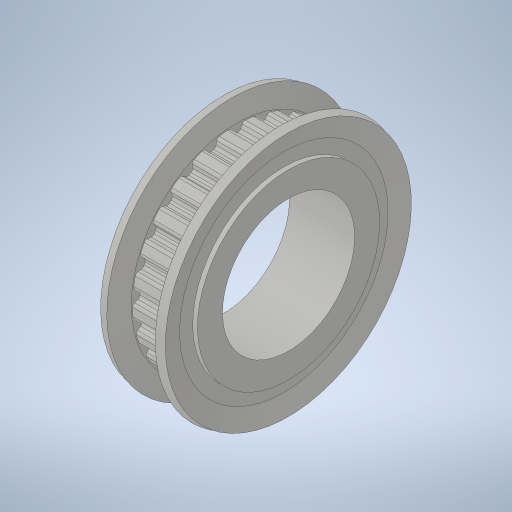
# Autodesk Inventor part: ATP25XL025-A-HUK_a
Saved by Autodesk Inventor 2023.1 (Build 271208000, 208)
## iProperties
Created: 2022-11-04
Part Number: ATP25XL025-A-HUK_a
Material: Generic
Catalog Web Link: www.cadenas.de
Description: ATP_ _XL025, ATP_ _XL031, ATP_ _ XL037, ATP_ _XL050, BTP_ _XL025, BTP_ _XL031, BTP_ _XL037, BTP_ _XL050, KTP_ _XL025, KTP_ _XL031, KTP_ _ XL037, KTP_ _XL050, NTP_ _XL025, NTP_ _XL031, NTP_ _ XL037, NTP_ _XL050, MTP_ _XL025, MTP_ _ XL037, MTP_ _XL050, MTPB_ _XL025, MTPB_ _ XL037, MTPB_ _XL050, MTPP_ _XL025, MTPP_ _ XL037, MTPP_ _XL050, STP_ _XL025, STP_ _ XL037, STP_ _XL050_aI-Timing Pulleys XL Type
Vendor: MISUMI
Document SubType Name: Modeling
Designer: psAdmin
Manufacturer: MISUMI
Mass: 10.0288 g
Surface Area: 66.7014 cm^2
Volume: 10.0288 cm^3
Density: 1 g/cm^3
Appearance: PSOLRGB-175-175-175
Category: PARTsolutions
Company: MISUMI
PSOL_IDENT_0: {$CADENAS_DATA/23d-libs/misumi/metric/51_timing_pulleys/timing_pulleys_inch/atp_xl_inch.prj},697 {VT
PSOL_IDENT_1: YP=3D},{NB=ATP25XL025-A-HUK_a},{LINA=ATP25XL025-A-HUK},{NN=ATP_ _XL025, ATP_ _XL031, ATP_ _ XL037, A
PSOL_IDENT_2: TP_ _XL050, BTP_ _XL025, BTP_ _XL031, BTP_ _XL037, BTP_ _XL050, KTP_ _XL025, KTP_ _XL031, KTP_ _ XL0
PSOL_IDENT_3: 37, KTP_ _XL050, NTP_ _XL025, NTP_ _XL031, NTP_ _ XL037, NTP_ _XL050, MTP_ _XL025, MTP_ _ XL037, MTP
PSOL_IDENT_4: _ _XL050, MTPB_ _XL025, MTPB_ _ XL037, MTPB_ _XL050, MTPP_ _XL025, MTPP_ _ XL037, MTPP_ _XL050, STP_
PSOL_IDENT_5: _XL025, STP_ _ XL037, STP_ _XL050_aI},{DATE=08.06.2021 06:34:01},{GEOMDATE=19.11.2018 09:46:42},{VE
PSOL_IDENT_6: RSION=},{LINEID=120},{WBVAR=MATP,ST,TNW,PS,SHS,DD,ALT2,M,QSC,QFC,QTC,ALT7,K,KSC,KFC,KTC,ALT1,ALT3,AL
PSOL_IDENT_7: T4,ALT5,FC,ALT6,TPC,ALT8,BC,ALT9,SLH},{WBNUMERIC=DD,QSC,QFC,QTC,K,KSC,KFC,KTC,FC,TPC,BC,SLH}  {NB=AT
PSOL_IDENT_8: P25XL025-A-HUK_a},{LINA=ATP25XL025-A-HUK},{KT=DUMMY},{PN=ATP25XL025-A-HUK},{TYPE=ATP},{MATP=ATP},{MA
PSOL_IDENT_9: TPA='ATP','2017 Aluminum Alloy (Duralumin)','MTP','1045 Carbon Steel','STP','304 Stainless Steel'},{
PSOL_IDENT_10: MATF=5052 Aluminum Alloy},{ST=CA},{HARD=-},{STA= 'CA' , 'Clear Anodize' , 'BA','Black Anodize','HAT'
PSOL_IDENT_11: ,'Hard Clear Anodize','ENP' , 'Electroless Nickel Plating' },{NT=25},{TNW=XL025},{TNW1=      'XL025'
PSOL_IDENT_12: ,'XL031','XL037','XL050'                            },{BW=6.4mm (1/4inch)},{A=7.5},{W=12.5},{L=21},{
PSOL_IDENT_13: PS=A},{PSA='A','B'},{SHS=H},{SHS1= 'H','Inch Round Hole', 'P','Inch Round Hole + Tap','N','Inch ANSI
PSOL_IDENT_14: Key Groove Hole'},{SHS2=-HUK},{SHSA= 'H','Inch Round Hole', 'P','Inch Round Hole + Tap','N','Inch A
PSOL_IDENT_15: NSI Key Groove Hole'},{SHSB= 'H','Inch Round Hole', 'P','Inch Round Hole + Tap','N','Inch ANSI Key G
PSOL_IDENT_16: roove Hole'},{DD=1},{DDINCH=25.4},{DD1=0.3750,0.5,0.625,0.75,0.8750,1},{DDH=0.3750,0.5,0.625,0.75,0.
PSOL_IDENT_17: 8750,1},{DDP=0.3750,0.5,0.625,0.75},{DDN=0.3750,0.5,0.625,0.75},{DDNK=10},{DDC=10,12,15,16,18,19,20}
PSOL_IDENT_18: ,{DDV=[8:25/1]},{DDF=[8:24/1]},{DDY=[8:25/1]},{DD635=25},{Z=0},{Z1=0},{ZQRMIN=28},{ZMAX=27},{ZA=0},{
PSOL_IDENT_19: ZB=0},{ZAB=},{J=0},{JA=0},{JMAX=10.5},{JAB=},{QRMAX=27},{Q=0},{Q1=0},{Q2=},{R=0},{R1=0},{R2=},{S=0},
PSOL_IDENT_20: {S1=0},{S2=},{SMAX=6.5},{T=0},{T1=0},{T2=},{TMAX=8},{PD=40.43},{OD=39.92},{D=0},{DB=30},{F=48},{E=35
PSOL_IDENT_21: },{DE=35},{BJS9=0},{TTTI=0},{TTT=0},{AC=-},{NDM=6.000},{WL=12.5},{ALT2=},{ALT2A='','N/A'},{QMIN=32},
PSOL_IDENT_22: {QMAX=28},{M=-},{MA= '-' },{MAA=},{NDMALT=0.000},{QSC=0},{QSCA=0},{QSCAA=},{QFC=0},{QFCA=0},{QFCAA=}
PSOL_IDENT_23: ,{QTC=0},{QTCA=0},{QTCAA=},{QCMIN=29},{QCMAX=31},{QC=0},{ALT7=},{ALT7A='','N/A'},{ALT71=1},{ALT72=1}
PSOL_IDENT_24: ,{ALT73=1},{K=0.0},{KSC=0},{KSCA=  [0:0]       },{KSCAA=},{KFC=0},{KFCA=  [0:0]       },{KFCAA=},{KT
PSOL_IDENT_25: C=0},{KTCA=  [0:0]       },{KTCAA=},{KC=0},{KCMIN=30},{KCMAX=31},{KA=0},{KMAX=0.0},{KPN=},{ALT1=},{A
PSOL_IDENT_26: LT1A='','N/A'},{ALT3=},{ALT4=},{ALT4A= '', 'w/o Flange Attached on One Side Only', '-RFC'  , 'with R
PSOL_IDENT_27: FC (Flange Attached on The hub Side Only)', '-LFC'  , 'with LFC (Flange Attached on The Opposite Sid
PSOL_IDENT_28: e Only)' },{ALT5=},{ALT5A='','w/o FC (Flange Cut)','-FC','with FC (Flange Cut)'},{FC=0.0},{ODAINT=39
PSOL_IDENT_29: },{FCMIN=41.0},{FCMAX=46.0},{FCA=0},{FCAA=},{ALFA=25},{ZUB=1.270},{TT=0.5},{TAP1=21.000},{TAP2=0.000
PSOL_IDENT_30: },{TAP=0.000},{MM=4.5},{ALT6=},{ALT6A=         '','N/A'},{TPC=0},{TPCA=           0,'N/A'         },
PSOL_IDENT_31: {TPCAA=},{ALT8=},{ALT8A=   '','N/A'                         },{BC=0.0},{BCCA=0},{BCCAMIN=3},{BCPLANE=
PSOL_IDENT_32: 6.25},{BCCAMAX=8.5},{BCAA=},{TMP=},{KTT=7.76},{KYY=12.2},{PLANE=12.5},{TIF=1},{RUPE=1},{ALT9=},{ALT9
PSOL_IDENT_33: A= '','N/A' },{SLH=0},{SLHA=0},{SLHPN=},{LS=0},{WS=6},{SL=19.96},{SL2=19.96},{ANG=115.2},{SCREWALG=2
PSOL_IDENT_34: },{WLBC=12.5},{DDPN=K},{BBINCH=6.25},{KMAXALG=25.5}
NB: ATP25XL025-A-HUK_a
NN: ATP_ _XL025, ATP_ _XL031, ATP_ _ XL037, ATP_ _XL050, BTP_ _XL025, BTP_ _XL031, BTP_ _XL037, BTP_ _XL050, KTP_ _XL025, KTP_ _XL031, KTP_ _ XL037, KTP_ _XL050, NTP_ _XL025, NTP_ _XL031, NTP_ _ XL037, NTP_ _XL050, MTP_ _XL025, MTP_ _ XL037, MTP_ _XL050, MTPB_ _XL025, MTPB_ _ XL037, MTPB_ _XL050, MTPP_ _XL025, MTPP_ _ XL037, MTPP_ _XL050, STP_ _XL025, STP_ _ XL037, STP_ _XL050_aI
NT: 25
NBSYN: $PN._a
LINA: ATP25XL025-A-HUK
CATALOG: Misumi
PN: ATP25XL025-A-HUK
MATP: 2017 Aluminum Alloy (Duralumin)
MATF: 5052 Aluminum Alloy
ST: Clear Anodize
HARD: -
TNW: XL025
BW: 6.4mm (1/4inch)
A: 7.5
W: 12.5
L: 21
PS: A
SHS: Inch Round Hole
DD: 1
PD: 40.43
OD: 39.92
D: 0
F: 48
E: 35
AC: -
ALT2: N/A
M: -
QSC: 0
QFC: 0
QTC: 0
ALT7: N/A
K: 0
KSC: 0
KFC: 0
KTC: 0
ALT1: N/A
ALT3: w/o NFC (Flange not Attached)
ALT4: w/o Flange Attached on One Side Only
ALT5: w/o FC (Flange Cut)
FC: 0
ALT6: N/A
TPC: N/A
ALT8: N/A
BC: 0
ALT9: N/A
SLH: 0
SUPPLIER: MISUMI
ARTICLENO: ATP25XL025-A-HUK_a
BOMINFO: ATP25XL025-A-HUK
CREATOR: CADENAS GmbH
Title: ATP25XL025-A-HUK
Author: Cadenas PARTsolutions
Comments: Timing Pulleys XL Type
Autodesk Inventor part; units mm, degrees
ref_plane "YZ Plane" through (0, 0, 0) normal (1, 0, 0) x (0, 1, 0)
ref_plane "XZ Plane" through (0, 0, 0) normal (0, 1, 0) x (-1, 0, 0)
ref_plane "XY Plane" through (0, 0, 0) normal (0, 0, 1) x (1, 0, 0)
sketch "Sketch_5" plane through (0, 0, 0) normal (0, 0, 1) x (1, 0, 0)
  line L0 (21, 0) -> (0, 0)
  line L1 (0, 12.7) -> (12.5, 12.7)
  line L2 (12.5, 12.7) -> (12.5, 17.5)
  line L3 (12.5, 17.5) -> (11.6, 17.5)
  line L4 (11.6, 17.5) -> (11.6, 20.0274)
  line L5 (11.6, 20.0274) -> (12.4566, 23.6299)
  line L6 (12.4566, 23.6299) -> (10.9, 24)
  line L7 (10.9, 24) -> (10, 20.215)
  line L8 (10, 20.215) -> (10, 19.96)
  line L9 (10, 19.96) -> (2.5, 19.96)
  line L10 (2.5, 19.96) -> (2.5, 20.215)
  line L11 (2.5, 20.215) -> (1.6, 24)
  line L12 (1.6, 24) -> (0.0434, 23.6299)
  line L13 (0.0434, 23.6299) -> (0.9, 20.0274)
  line L14 (0.9, 20.0274) -> (0.9, 17.5)
  line L15 (0.9, 17.5) -> (0, 17.5)
  line L16 (0, 17.5) -> (0, 12.7)
  constraints: 34 end point
revolve "Revolution1" add sketch "Sketch_5" angle 360 about axis through (21, 0, 0) along (1, 0, 0)
sketch "Sketch_2" plane through (2.5, 0, 0) normal (1, 0, 0) x (0, 0, -1)
  line L0 (-1.7007, 26.6133) -> (-1.7007, 19.8874)
  arc A0 (-1.0959, 19.5374) -> (-1.7007, 19.8874) centre (-1.6487, 19.2796) ccw
  line L1 (-1.0959, 19.5374) -> (-0.8035, 18.9106)
  arc A1 (-0.8035, 18.9106) -> (-0.2427, 18.5584) centre (-0.2507, 19.1684) ccw
  arc A2 (0.2427, 18.5584) -> (-0.2427, 18.5584) centre (0, 0) ccw
  arc A3 (0.2427, 18.5584) -> (0.8035, 18.9106) centre (0.2507, 19.1684) ccw
  line L2 (0.8035, 18.9106) -> (1.0959, 19.5374)
  arc A4 (1.7007, 19.8874) -> (1.0959, 19.5374) centre (1.6487, 19.2796) ccw
  line L3 (1.7007, 19.8874) -> (1.7007, 26.6133)
  line L4 (1.7007, 26.6133) -> (-1.7007, 26.6133)
  constraints: 10 end point, 10 point on circle, 5 centre point
extrude "Extrusion1" cut sketch "Sketch_2" along normal blind 7.5
pattern_circular "Circular Pattern1" count 25 over 360 about axis through (2.5, 0, 0) along (1, 0, 0) of "Extrusion1"
ref_plane "to_s1_XY" through (6.25, 19.96, 0) normal (0, 1, 0) x (1, 0, 0)
ref_plane "to_s1_YZ" through (6.25, 19.96, 0) normal (1, 0, 0) x (0, 0, -1)
ref_plane "to_s1_ZX" through (6.25, 19.96, 0) normal (0, 0, -1) x (0, 1, 0)
ref_plane "to_s2_XY" through (6.25, -8.4986, -18.0603) normal (0, -0.4257793, -0.9048271) x (1, 0, 0)
ref_plane "to_s2_YZ" through (6.25, -8.4986, -18.0603) normal (1, 0, 0) x (0, -0.9048271, 0.4257793)
ref_plane "to_s2_ZX" through (6.25, -8.4986, -18.0603) normal (0, -0.9048271, 0.4257793) x (0, -0.4257793, -0.9048271)
body "Solid1"
